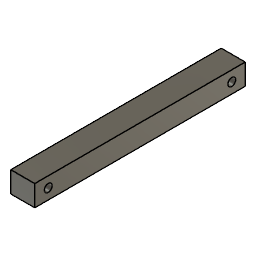
Dump Link (Autodesk Fusion 360 design; units mm, degrees)
Autodesk Fusion 360 part; units mm, degrees
sketch "Sketch1" plane through (0, 0, 0) normal (1, 0, 0) x (0, 1, 0)
  circle A0 centre (0, 0) radius 2.6
  circle A1 centre (122, 0) radius 2.6
  line L0 (-9, 7) -> (131, 7)
  line L1 (131, 7) -> (131, -7)
  line L2 (131, -7) -> (-9, -7)
  line L3 (-9, -7) -> (-9, 7)
  dimension "d1" = 5.2
  dimension "d3" = 5.2
  constraint coincident A0.centre origin
  constraint horizontal L0
  constraint vertical L1
  constraint horizontal L2
  constraint vertical L3
  measures "d1" diameter of A0
  measures "d3" diameter of A1
extrude "Extrude1" add sketch "Sketch1" along normal mid plane 16
